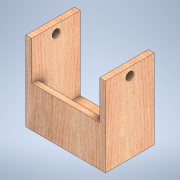
# Autodesk Inventor part: woodForkAssembly02
Saved by Autodesk Inventor 2022.2 (Build 262287000, 287)
## iProperties
Created: 2020-07-02
Part Number: woodForkAssembly02
Material: Wood (Birch)
Document SubType Name: Modeling
Designer: robst
Density: 0.55 g/cm^3
Appearance: Birch - Natural Polished
Mass: 1433.83 g
Surface Area: 3055.89 cm^2
Volume: 2606.97 cm^3
Author: robst
Autodesk Inventor part; units mm, degrees
ref_plane "YZ Plane" through (0, 0, 0) normal (1, 0, 0) x (0, 1, 0)
ref_plane "XZ Plane" through (0, 0, 0) normal (0, 1, 0) x (-1, 0, 0)
ref_plane "XY Plane" through (0, 0, 0) normal (0, 0, 1) x (1, 0, 0)
sketch "Sketch1" plane through (0, 0, 0) normal (0, 1, 0) x (-1, 0, 0)
  line L0 (130.175, 79.375) -> (-130.175, 79.375)
  line L1 (-130.175, 79.375) -> (-130.175, -79.375)
  line L2 (-130.175, -79.375) -> (130.175, -79.375)
  line L3 (130.175, -79.375) -> (130.175, 79.375)
  line L4 (130.175, 79.375) -> (-130.175, -79.375) construction
  line L5 (-130.175, 79.375) -> (130.175, -79.375) construction
  point P0 (0, 0)
  dimension "d0" = 260.35
  dimension "d1" = 158.75
  constraints: 12 end point, 2 midpoint, 2 parallel, 1 horizontal, 1 perpendicular
  measures "d0" distance of L0.start L0.end
  measures "d1" distance of L1.end L0.end
extrude "Base" add sketch "Sketch1" against normal blind 19.05
sketch "Sketch2" plane through (0, 0, 0) normal (0, 1, 0) x (1, 0, 0)
  line L0 (-130.175, -79.375) -> (-130.175, 79.375) projected
  line L1 (-130.175, 79.375) -> (-111.125, 79.375)
  line L2 (-111.125, 79.375) -> (-111.125, -79.375)
  line L3 (-111.125, -79.375) -> (-130.175, -79.375)
  line L4 (-130.175, -79.375) -> (-130.175, 79.375)
  line L5 (130.175, 79.375) -> (130.175, -79.375) projected
  line L6 (130.175, -79.375) -> (-130.175, -79.375) projected
  line L7 (130.175, 79.375) -> (111.125, 79.375)
  line L8 (111.125, 79.375) -> (111.125, -79.375)
  line L9 (111.125, -79.375) -> (130.175, -79.375)
  line L10 (130.175, -79.375) -> (130.175, 79.375)
  line L11 (-130.175, -79.375) -> (130.175, -79.375) projected
  point P0 (0, 0)
  dimension "d4" = 19.05
  constraints: 16 end point, 4 parallel, 2 collinear, 2 horizontal, 2 perpendicular, 1 point on line
  measures "d4" distance of L0.end L1.end
extrude "Sides" add sketch "Sketch2" along normal blind 241.3
sketch "Sketch3" plane through (0, 0, 0) normal (0, 1, 0) x (1, 0, 0)
  line L0 (-130.175, -79.375) -> (-111.125, -79.375) projected
  line L1 (111.125, 79.375) -> (111.125, -79.375) projected
  line L2 (-111.125, -79.375) -> (111.125, -79.375)
  line L3 (111.125, -79.375) -> (111.125, -60.325)
  line L4 (111.125, -60.325) -> (-111.125, -60.325)
  line L5 (-111.125, -60.325) -> (-111.125, -79.375)
  point P0 (0, 0)
  point P1 (111.125, -79.375)
  dimension "d7" = 19.05
  constraints: 8 end point, 2 parallel, 1 horizontal, 1 perpendicular, 1 point on line
  measures "d7" distance of L4.end L0.end
extrude "FrontPiece" add sketch "Sketch3" along normal blind 114.3
sketch "Sketch5" plane through (130.175, -19.05, 79.375) normal (1, 0, 0) x (0, 0, -1)
  line L0 (158.75, 260.35) -> (0, 260.35) construction
  line L1 (79.375, 260.35) -> (79.375, 0) construction
  line L2 (0, 0) -> (158.75, 0) construction
  line L3 (19.05, 19.05) -> (158.75, 19.05) projected
  point P0 (79.375, 19.05)
  point P1 (79.375, 234.95)
  dimension "d23" = 215.9
  constraints: 2 end point, 2 midpoint, 1 point on line
  measures "d23" distance from line of point (79.375, 234.95) L3
hole "HoleForSides" at (130.175, 215.9, 0) direction (-1, 0, 0) diameter 25.908 end through all
sketch "Sketch8" plane through (0, 0, 0) normal (0, 1, 0) x (1, 0, 0)
  circle A0 centre (0, 0) radius 15.875
  dimension "d27" = 31.75
  constraints: 1 centre point, 1 coincident
  measures "d27" diameter of A0
extrude "BottomHole" cut sketch "Sketch8" against normal through all
equation "\"d0\" = interiorWidth + 2 * woodThickness"
equation "\"d1\" = partDepth"
equation "\"d2\" = woodThickness"
equation "\"d4\" = woodThickness"
equation "\"d5\" = totalHeight - woodThickness"
equation "\"d7\" = woodThickness"
equation "\"d8\" = supportBoardHeight"
equation "\"d23\" = holeCenter"
equation "\"d13\" = holeDiameter"
equation "\"interiorWidth\" = 222.25"
equation "\"woodThickness\" = 19.05"
equation "\"holeCenter\" = 215.9"
equation "\"supportBoardHeight\" = 114.3"
equation "\"holeDiameter\" = 25.908"
equation "\"partDepth\" = 158.75"
equation "\"totalHeight\" = 260.35"
body "Solid1"
